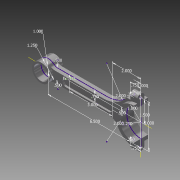
# Autodesk Inventor part: HW 7 Part 3
Saved by Autodesk Inventor 2015 (Build 190159000, 159)
## iProperties
Created: 2016-02-22
Part Number: HW 7 Part 3
Material: Steel, Carbon
Document SubType Name: Modeling
Designer: melissa.roth
Density: 7.85 g/cm^3
Appearance: Semi-Polished
Mass: 406.16 g
Surface Area: 217.298 cm^2
Volume: 51.7401 cm^3
Author: melissa.roth
Autodesk Inventor part; units mm, degrees
ref_plane "YZ Plane" through (0, 0, 0) normal (1, 0, 0) x (0, 1, 0)
ref_plane "XZ Plane" through (0, 0, 0) normal (0, 1, 0) x (-1, 0, 0)
ref_plane "XY Plane" through (0, 0, 0) normal (0, 0, 1) x (1, 0, 0)
sketch "Sketch1" plane through (0, 0, 0) normal (0, 0, 1) x (1, 0, 0)
  arc A0 (0, 25.4) -> (0, -25.4) centre (0, 0) ccw
  arc A1 (0, 31.75) -> (0, -31.75) centre (0, 0) ccw
  line L0 (0, 31.75) -> (0, 25.4)
  line L1 (0, 7.578) -> (0, -31.75)
  line L2 (0, 31.75) -> (0, 38.1)
  line L3 (0, 38.1) -> (-12.7, 38.1)
  line L4 (-12.7, 38.1) -> (-12.7, 31.75)
  line L5 (-12.7, 31.75) -> (-19.05, 31.75)
  line L6 (0, -31.75) -> (0, -38.1)
  line L7 (0, -38.1) -> (-12.7, -38.1)
  line L8 (-12.7, -38.1) -> (-12.7, -31.75)
  line L9 (-12.7, -31.75) -> (-19.05, -31.75)
  line L10 (-61.0513, 9.525) -> (-147.1395, 9.525)
  circle A2 centre (-165.1, 0) radius 12.7
  circle A3 centre (-165.1, 0) radius 15.875
  line L11 (-147.1395, -9.525) -> (-61.0513, -9.525)
  arc A4 (-19.05, -31.75) -> (-61.0513, -9.525) centre (-61.0513, -60.325) ccw
  arc A5 (-61.0513, 9.525) -> (-19.05, 31.75) centre (-61.0513, 60.325) ccw
  arc A6 (-155.1219, 12.3472) -> (-147.1395, 9.525) centre (-147.1395, 22.225) ccw
  arc A7 (-147.1395, -9.525) -> (-155.1219, -12.3472) centre (-147.1395, -22.225) ccw
  line L12 (-127, 0) -> (-50.8, 0) construction
  line L13 (-127, 6.35) -> (-50.8, 6.35)
  line L14 (-50.8, -6.35) -> (-127, -6.35)
  arc A8 (-127, 6.35) -> (-127, -6.35) centre (-127, 0) ccw
  arc A9 (-50.8, -6.35) -> (-50.8, 6.35) centre (-50.8, 0) ccw
  line L15 (0, -25.4) -> (0, -31.75)
  line L16 (0, 31.75) -> (0, 25.4)
  point P0 (-88.9, 0)
  dimension "d0" = 165.1
  dimension "d1" = 25.4
  dimension "d2" = 31.75
  dimension "d3" = 76.2
  dimension "d4" = 50.8
  dimension "d5" = 50.8
  dimension "d6" = 12.7
  dimension "d7" = 12.7
  dimension "d8" = 31.75
  dimension "d9" = 25.4
  dimension "d10" = 6.35
  dimension "d11" = 6.35
  dimension "d12" = 12.7
  dimension "d14" = 19.05
  dimension "d16" = 19.05
  dimension "d17" = 9.525
  dimension "d18" = 38.1
  dimension "d21" = 19.05
  dimension "d22" = 12.7
  dimension "d23" = 76.2
  dimension "d24" = 50.8
  dimension "d37" = 0
  constraints: 36 end point, 18 point on circle, 10 centre point, 10 tangent, 6 perpendicular, 4 collinear, 4 vertical, 3 coincident, 3 horizontal, 1 horizontal alignment, 1 midpoint, 1 parallel
  measures "d0" distance of point (0, 0) A2.centre
  measures "d1" radius of A0
  measures "d2" radius of A1
  measures "d3" distance of L6.end L2.end
  measures "d4" radius of A5
  measures "d5" radius of A4
  measures "d6" radius of A7
  measures "d7" radius of A6
  measures "d8" diameter of A3
  measures "d9" diameter of A2
  measures "d10" distance of L3.end L4.end
  measures "d11" distance of L7.end L8.end
  measures "d12" distance of L2.end L3.end
  measures "d14" horizontal distance of L2.end L5.end
  measures "d16" distance between parallel lines of L11 L10
  measures "d17" distance from line of point (0, 0) L10
  measures "d18" distance from line of point (0, 0) L3
  measures "d21" horizontal distance of L6.end L9.end
  measures "d22" distance between parallel lines of L14 L13
  measures "d23" distance of L12.end L12.start
  measures "d24" horizontal distance of L0.end L12.end
  measures "d37" distance from line of point (0, 0) L0
extrude "Extrusion1" add sketch "Sketch1" along normal mid plane 6.35 contours A0 L1 A1 L0 | A1 L6 L7 L8 L9 A4 L11 A7 A3 A6 L10 A5 L5 L4 L3 L2 | A3 | L13 A9 L14 A8
extrude "Extrusion2" add sketch "Sketch1" along normal mid plane 25.4 contours A0 L1 A1 L0 | A3
extrude "Extrusion3" add sketch "Sketch1" along normal mid plane 12.7 contours A1 L6 L7 L8 L9 A4 L11 A7 A3 A6 L10 A5 L5 L4 L3 L2
sketch "Sketch2" plane through (0, 0, 0) normal (1, 0, 0) x (0, 1, 0)
  line L0 (38.1, -6.35) -> (38.1, 6.35) projected
  circle A0 centre (38.1, 0) radius 3.175
  circle A1 centre (-38.1, 0) radius 3.175
  arc A2 (38.1, -6.35) -> (38.1, 6.35) centre (38.1, 0) ccw
  arc A3 (-38.1, 6.35) -> (-38.1, -6.35) centre (-38.1, 0) ccw
  line L1 (38.1, 6.35) -> (38.1, -6.35)
  line L2 (-38.1, 6.35) -> (-38.1, -6.35)
  line L3 (-38.1, -6.35) -> (-38.1, 6.35) projected
  point P0 (0, 0)
  dimension "d31" = 6.35
  dimension "d32" = 6.35
  constraints: 4 centre point, 4 end point, 4 point on circle, 2 coincident, 2 collinear, 1 midpoint
  measures "d31" diameter of A0
  measures "d32" diameter of A1
extrude "Extrusion4" add sketch "Sketch2" against normal blind 12.7 contours L0 A0 A2 | L0 A0 | L2 A1 | A1 L2 A3 picked at (40.0502, 0.2355) picked at (-38.971, -0.6012)
extrude "Extrusion5" cut sketch "Sketch2" against normal blind 12.7 contours A0 L0 | L0 A0 | A1 L2 | L2 A1
equation "\"d17\" = 0.5 * d16"
equation "\"d32\" = d31"
body "Solid1"
